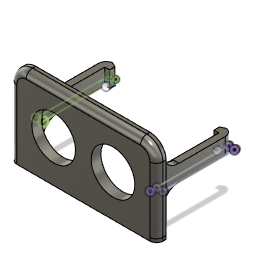
R1200GS foglight switch replacement v11 (Autodesk Fusion 360 design; units mm, degrees)
Autodesk Fusion 360 part; units mm, degrees
sketch "Front panel" plane through (0, 0, 0) normal (0, 0, 1) x (1, 0, 0)
  line L0 (41.5, -22) -> (0, -22)
  line L1 (-2.0009, 2.3789) -> (43.4991, 2.3789)
  line L2 (38.5, -8.5) -> (38.5, -13.5)
  line L3 (41.5, -13.5) -> (41.5, -8.5)
  line L4 (-1.25, -23) -> (-1.25, -13)
  line L5 (-1.25, -13) -> (0, -13)
  line L6 (0, -13) -> (0, -22)
  line L7 (7.0062, 0) -> (7.0062, 1.25)
  line L8 (-1.2476, -6.6211) -> (0.0024, -6.6211)
  line L9 (34.5075, -0.0004) -> (34.5074, 1.2496)
  line L10 (42.75, -6.6211) -> (41.5, -6.6211)
  line L11 (42.75, -23) -> (42.75, -13)
  line L12 (42.75, -13) -> (41.5, -13)
  line L13 (41.5, -13) -> (41.5, -22)
  line L14 (3, -8.5) -> (3, -13.5)
  line L15 (0, -13.5) -> (0, -8.5)
  arc A0 (7.0062, 0) -> (0.0024, -6.6211) centre (7.0103, -7.0192) ccw
  arc A1 (41.5, -6.6211) -> (34.5075, -0.0004) centre (34.8695, -6.6211) ccw
  line L16 (1, -8.5) -> (1, -13.5)
  line L17 (40.5, -8.5) -> (40.5, -13.5)
  line L18 (42.75, -23) -> (41.5, -23)
  line L19 (41.5, -23) -> (41.5, -22)
  line L20 (0, -22) -> (0, -23)
  line L21 (-1.25, -23) -> (0, -23)
  arc A2 (42.75, -3.1248) -> (38.625, 1.25) centre (38.477, -3.0217) ccw
  arc A3 (2.8785, 1.25) -> (-1.2549, -3.1346) centre (3.1277, -3.1255) ccw
  line L22 (2.8785, 1.25) -> (7.0062, 1.25)
  line L23 (-1.2549, -3.1346) -> (-1.2476, -6.6211)
  line L24 (42.75, -3.1248) -> (42.75, -6.6211)
  line L25 (38.625, 1.25) -> (34.5074, 1.2496)
  circle A4 centre (11.4915, -11.1211) radius 6.8
  circle A5 centre (29.9797, -11.1211) radius 6.8
  line L26 (41.5, -6.6211) -> (41.5, -13)
  line L27 (0.0024, -6.6211) -> (0, -8.5)
  line L28 (43.4795, -23) -> (42.75, -23)
  line L29 (41.5, -23) -> (0, -23)
  line L30 (-1.25, -23) -> (-2.0085, -23)
  line L31 (-2.0085, -2.6211) -> (-2.0085, -23)
  line L32 (43.4798, -2.621) -> (43.4795, -23)
  line L33 (40.5, -8.5) -> (38.5, -8.5)
  line L34 (40.5, -13.5) -> (38.5, -13.5)
  line L35 (3, -8.5) -> (1, -8.5)
  line L36 (1, -13.5) -> (3, -13.5)
  line L37 (3.0215, -3.8994) -> (3.0215, -20.7559)
  line L38 (3.0215, -20.7559) -> (38.6674, -20.7559)
  line L39 (38.6674, -20.7559) -> (38.6674, -3.8994)
  arc A6 (43.4798, -2.621) -> (38.4991, 2.3789) centre (38.4799, -2.621) ccw
  arc A7 (2.9991, 2.3789) -> (-2.0085, -2.6211) centre (2.9491, -2.5787) ccw
  line L40 (38.6674, -3.8994) -> (38.6674, -1.186)
  line L41 (3.0215, -3.8994) -> (3.0215, -1.2435)
  dimension "d2" = 22
  dimension "d3" = 45.5
  dimension "d10" = 3
  dimension "d11" = 5
  dimension "d24" = 10
  dimension "d25" = 10
  dimension "d26" = 5
  dimension "d27" = 3
  dimension "d46" = 9
  dimension "d49" = 9
  dimension "d50" = 1.25
  dimension "d51" = 1.25
  dimension "d52" = 1.25
  dimension "d53" = 1.25
  dimension "d56" = 1
  dimension "d61" = 1
  dimension "d62" = 1
  dimension "d63" = 1.25
  dimension "d64" = 1.25
  dimension "d66" = 5
  dimension "d68" = 5
  dimension "d71" = 13.6
  dimension "d72" = 13.6
  dimension "d73" = 13.5
  dimension "d74" = 13.5
  dimension "d77" = 13.5
  dimension "d78" = 13.5
  dimension "d79" = 5
  dimension "d81" = 5
  constraint horizontal L0
  constraint horizontal L1
  constraint vertical L2
  constraint vertical L3
  constraint vertical L4
  constraint horizontal L5
  constraint vertical L6
  constraint vertical L11
  constraint horizontal L12
  constraint vertical L13
  constraint vertical L14
  constraint vertical L15
  constraint perpendicular L13 L18
  constraint perpendicular L0 L19
  constraint perpendicular L0 L20
  constraint perpendicular L4 L21
  constraint perpendicular L7 L22
  constraint tangent A3 L23
  constraint perpendicular L10 L24
  constraint perpendicular L9 L25
  constraint tangent A1 L26
  constraint perpendicular L11 L28
  constraint perpendicular L2 L33
  constraint perpendicular L2 L34
  constraint perpendicular L16 L35
  constraint perpendicular L14 L36
  constraint vertical L37
  constraint horizontal L38
  constraint vertical L39
  constraint tangent L32 A6
  constraint coincident L1 A6.end
  constraint vertical L31
  constraint tangent A3 A7
  constraint coincident L1 A7.start
  constraint coincident A1 L40.end
  constraint vertical L40
  constraint coincident A0 L41.end
  constraint vertical L41
  measures "d2" distance of origin L0.end
  measures "d3" distance of L1.start L1.end
  measures "d10" distance of L3.end L2.start
  measures "d11" distance of L2.start L2.end
  measures "d24" distance of L11.start L11.end
  measures "d25" distance of L4.start L4.end
  measures "d26" distance of L14.start L14.end
  measures "d27" distance of L15.end L14.start
  measures "d46" distance of L1 L8
  measures "d49" distance of L1 L10
  measures "d50" distance of L8.start L8.end
  measures "d51" distance of L7.start L7.end
  measures "d52" distance of L10.start L10.end
  measures "d53" distance of L9.start L9.end
  measures "d56" distance of L3 L17
  measures "d61" distance of L0.start L18
  measures "d62" distance of L0 L21
  measures "d63" distance of L4.start L20.end
  measures "d64" distance of L11.start L18.end
  measures "d66" distance of L1.start L31.start
  measures "d68" distance of L1.end L32.start
  measures "d71" diameter of A4
  measures "d72" diameter of A5
  measures "d73" distance of L1 A5.centre
  measures "d74" distance of L1 A4.centre
  measures "d77" distance of A5.centre L32
  measures "d78" distance of A4.centre L31
  measures "d79" distance of L1.end A6.end
  measures "d81" distance of L1.start A7.start
extrude "Extrude1" add sketch "Front panel" along normal blind 2 contours L0 L19 L20 L29 | L0 L3 L6 L13 L15 A0 A1 L17 L26 L27 L33 L34 L37 L38 L39 L40 L41 | L1 L2 L3 L4 L5 L7 L8 L9 L10 L11 L12 L15 A0 A1 A2 A3 L22 L23 L24 L25 L26 L27 L28 L30 L31 L32 L33 L34 L37 L38 L39 A6 A7 L40 L41 | L2 L33 L34 L39 | L17 L33 L34 L39 | L14 L16 L35 L36
extrude "Extrude2" add sketch "Front panel" against normal blind 2 contours L0 L3 L6 L13 L15 A0 A1 L17 L26 L27 L33 L34 L37 L38 L39 L40 L41 | L2 L33 L34 L39 | L17 L33 L34 L39 | L14 L16 L35 L36
extrude "Extrude4" add sketch "Front panel" against normal blind 24.3 contours L2 L33 L34 L39 | L17 L33 L34 L39 | L14 L16 L35 L36
sketch "Leg barbs" plane through (0, -13.5, 0) normal (0, -1, 0) x (1, 0, 0)
  line L0 (38.5, -2) -> (38.5, -24.8)
  line L1 (38.5, -24.8) -> (40.5, -24.8)
  line L2 (38.5, -21.4) -> (37, -21.4)
  line L3 (3, -2) -> (3, -24.8)
  line L4 (3, -21.4) -> (4.5, -21.4)
  line L5 (3, -24.8) -> (1, -24.8)
  line L6 (1, -24.8) -> (4.5, -23.0579)
  line L7 (4.5, -23.0579) -> (4.5, -21.4)
  line L8 (37, -21.4) -> (37, -23.1052)
  line L9 (37, -23.1052) -> (40.5, -24.8)
  line L10 (40.5, -24.8) -> (40.5, -2)
  arc A0 (38.5, -23.8315) -> (40.5, -21.4) centre (38.0219, -21.4) ccw
  arc A1 (1, -21.4) -> (3, -23.8045) centre (3.4454, -21.4) ccw
  line L11 (1, -2) -> (1, -24.8)
  line L12 (40.5, -2) -> (38.5, -2)
  line L13 (40.5, -2) -> (38.6674, -2)
  line L14 (38.5, 0) -> (38.5, -24.3)
  line L15 (38.5, -24.3) -> (40.5, -24.3)
  line L16 (40.5, -24.3) -> (40.5, -2)
  line L17 (38.6674, 0) -> (38.5, 0)
  line L18 (38.6674, -2) -> (38.6674, 0)
  dimension "d34" = 1.5
  dimension "d35" = 3.4
  dimension "d37" = 3.4
  dimension "d54" = 1.5
  constraint coincident L0 L2.start
  constraint perpendicular L0 L2
  constraint coincident L3 L4.start
  constraint perpendicular L0 L4
  constraint coincident L1.end L9.end
  constraint coincident L5.end L6.start
  constraint perpendicular L4 L7
  constraint perpendicular L2 L8
  constraint tangent L10 A0
  constraint coincident L10 A0.end
  constraint coincident L9 A0.start
  constraint coincident L0 A0.start
  constraint tangent A1 L11
  constraint coincident L3 A1.end
  constraint coincident L6 A1.end
  constraint coincident A1.start L11
  measures "d34" distance of L2.start L2.end
  measures "d35" distance of L1 L2
  measures "d37" distance of L4 L5
  measures "d54" distance of L4.start L4.end
extrude "Extrude10" add sketch "Front panel" along normal blind 1 from surface at 2 contours L0 L19 L20 L29 | L0 L3 L6 L13 L15 A0 A1 L17 L26 L27 L33 L34 L37 L38 L39 L40 L41 | L3 L11 L12 L13 L18 L19 | L4 L5 L6 L15 L20 L21 | L1 L2 L3 L4 L5 L7 L8 L9 L10 L11 L12 L15 A0 A1 A2 A3 L22 L23 L24 L25 L26 L27 L28 L30 L31 L32 L33 L34 L37 L38 L39 A6 A7 L40 L41 | L9 L10 A1 A2 L24 L25 | L7 L8 A0 A3 L22 L23 | L2 L33 L34 L39 | L17 L33 L34 L39 | L14 L16 L35 L36
fillet "Fillet1" radius 2 5 edges at (20.6991, 2.3789, 3) (43.4797, -12.8105, 3) (42.0222, 0.9077, 3) (-2.0085, -12.8105, 3) (-0.5891, 0.8942, 3)
extrude "Extrude8" add sketch "Leg barbs" against normal blind 5 contours L0 L2 L8 L9 L14 | L3 L4 L6 L7
extrude "Extrude9" cut sketch "Leg barbs" against normal blind 5 contours L0 L9 L14 L15 | L9 L10 A0 L15 L16 | L0 L1 L9 L15 | L9 L10 L15 | L3 L5 L6 | L6 A1 L11
fillet "Fillet2" radius 5 3 edges at (39.5837, -8.5, -2) (2, -8.5, -2) (2, -13.5, -2)
fillet "Fillet2" radius 5 1 edges at (39.5837, -13.5, -2)
extrude "Extrude11" add 1 faces at (27.6667, -23, 0.6667) along direction (0, -1, 0) blind 1
equation "d4 = 27 mm"
equation "d8 = 5 mm"
equation "d11 = d8"
equation "d13 = 1.25 mm"
equation "d26 = d11"
equation "d37 = d35"
equation "d49 = d46"
equation "d50 = d13"
equation "d51 = d50"
equation "d52 = d50"
equation "d53 = d51"
equation "d54 = d34"
equation "d55 = 1 mm"
equation "d56 = d55"
equation "d73 = d4 / 2"
equation "d74 = d4 / 2"
